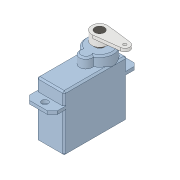
# Autodesk Inventor part: CW
Saved by Autodesk Inventor 2019 (Build 230136000, 136)
## iProperties
Created: 2022-04-05
Part Number: CW
Material: Generic
Document SubType Name: Modeling
Designer: solyo
Density: 1 g/cm^3
Appearance: Default
Mass: 3.44386 g
Surface Area: 17.9461 cm^2
Volume: 3.44386 cm^3
Author: solyo
Autodesk Inventor part; units mm, degrees
ref_plane "YZ Plane" through (0, 0, 0) normal (1, 0, 0) x (0, 1, 0)
ref_plane "XZ Plane" through (0, 0, 0) normal (0, 1, 0) x (-1, 0, 0)
ref_plane "XY Plane" through (0, 0, 0) normal (0, 0, 1) x (1, 0, 0)
sketch "Sketch1" plane through (0, 0, 0) normal (0, 1, 0) x (-1, 0, 0)
  line L0 (-4.375, -10) -> (4.375, -10)
  line L1 (4.375, -10) -> (4.375, 10)
  line L2 (4.375, 10) -> (-4.375, 10)
  line L3 (-4.375, 10) -> (-4.375, -10)
  line L4 (-4.375, -10) -> (4.375, 10) construction
  line L5 (4.375, -10) -> (-4.375, 10) construction
  point P0 (0, 0)
  dimension "d0" = 8.75
  dimension "d1" = 20
  constraints: 12 end point, 2 midpoint, 2 parallel, 1 horizontal, 1 perpendicular
  measures "d0" distance of L2.end L1.end
  measures "d1" distance of L1.end L0.end
extrude "Extrusion1" add sketch "Sketch1" along normal blind 17.7
ref_plane "Work Plane1" through (0, 12.7, 0) normal (0, -1, 0) x (1, 0, 0)
sketch "Sketch2" plane through (0, 12.7, 0) normal (0, -1, 0) x (1, 0, 0)
  line L0 (4.375, -10) -> (-4.375, -10) projected
  line L1 (4.375, -10) -> (-4.375, -10) projected
  line L2 (-4.375, -10) -> (-4.375, 10) projected
  line L3 (-4.375, 10) -> (4.375, 10) projected
  line L4 (4.375, 10) -> (4.375, -10) projected
  line L5 (-4.375, 13.75) -> (4.375, 13.75)
  line L6 (4.375, 13.75) -> (4.375, -13.75)
  line L7 (4.375, -13.75) -> (-4.375, -13.75)
  line L8 (-4.375, -13.75) -> (-4.375, 13.75)
  point P0 (0, 0)
  point P1 (0, 11.75)
  point P2 (0, -11.75)
  point P3 (0, -10)
  dimension "d5" = 23.5
  dimension "d6" = 2
  dimension "d7" = 2
  dimension "d8" = 11.75
  dimension "d9" = 11.75
  constraints: 8 end point, 4 vertical alignment, 2 parallel, 1 horizontal, 1 midpoint, 1 perpendicular
  measures "d5" distance of point (0, -11.75) point (0, 11.75)
  measures "d6" distance from line of point (0, -11.75) L7
  measures "d7" distance from line of L5 point (0, 11.75)
  measures "d8" distance of point (0, 0) point (0, -11.75)
  measures "d9" distance of point (0, 0) point (0, 11.75)
extrude "Extrusion2" add sketch "Sketch2" against normal blind 1 contours L6 L7 L8 L0 | L3 L8 L5 L6
chamfer "Chamfer1" distance 1.5 angle 45 4 edges at (4.375, 13.2, 13.75) (-4.375, 13.2, 13.75) (4.375, 13.2, -13.75) (-4.375, 13.2, -13.75)
hole "Hole1" at (0, 12.7, 11.75) at (0, 12.7, -11.75) direction (0, 1, 0) diameter 2 end through all
sketch "Sketch3" plane through (0, 17.7, 0) normal (0, 1, 0) x (1, 0, 0)
  circle A0 centre (0, 5.625) radius 4.375
  circle A1 centre (0, 1.25) radius 2
  line L0 (4.375, 10) -> (-4.375, 10) projected
  line L1 (-4.375, 10) -> (-4.375, -10) projected
  line L2 (-4.375, -10) -> (4.375, -10) projected
  line L3 (4.375, -10) -> (4.375, 10) projected
  circle A2 centre (0, 11.75) radius 1 projected
  point P0 (0, 0)
  dimension "d23" = 4
  constraints: 3 vertical alignment, 1 centre point, 1 horizontal, 1 vertical, 2 other
  measures "d23" diameter of A1
extrude "Extrusion3" add sketch "Sketch3" along normal blind 3.15 contours A0 A1 | A1 A0 | A0 A1
chamfer "Chamfer2" distance 0.5 angle 45 22 edges at (4.375, 15.7, 10) (-4.375, 15.7, 10) (-4.375, 6.35, 10) (4.375, 6.35, 10) (4.375, 6.35, -10) (4.375, 15.7, -10) (-4.375, 15.7, -10) (-4.375, 6.35, -10) (4.375, 17.7, 2.1875) (4.375, 17.7, -7.8125) (0, 13.7, -13.75) (-4.375, 17.7, 2.1875) (0, 17.7, 10) (4.375, 0, 0) (0, 0, 10) (-4.375, 0, 0) (0, 0, -10) (0, 20.85, 0.75) (0, 20.85, -10) (-4.375, 17.7, -7.8125) (-2.1875, 17.7, -10) (2.1875, 17.7, -10)
sketch "Sketch4" plane through (0, 20.85, 0) normal (0, 1, 0) x (1, 0, 0)
  arc A0 (1.3112, 1.9786) -> (-1.3112, 1.9786) centre (0, 5.625) ccw projected
  arc A1 (-1.3112, 1.9786) -> (1.3112, 1.9786) centre (0, 1.25) ccw projected
  circle A2 centre (0, 5.625) radius 1.5
  point P0 (0, 0)
  dimension "d31" = 3
  constraints: 1 centre point, 1 coincident
  measures "d31" diameter of A2
extrude "Extrusion4" add sketch "Sketch4" along normal blind 4 separate body contours A2
sketch "Sketch5" plane through (0, 24.85, -5.625) normal (0, 1, 0) x (1, 0, 0)
  circle A0 centre (0, 0) radius 1.5 projected
  arc A1 (2.4804, -0.3125) -> (-2.4804, -0.3125) centre (0, 0) ccw
  arc A2 (-1.4882, -8.1875) -> (1.4882, -8.1875) centre (0, -8) ccw
  line L0 (0, 0) -> (0, -23.0881) construction
  line L1 (0, -8) -> (0, 0) construction
  line L2 (1.4882, -8.1875) -> (2.4804, -0.3125)
  line L3 (-1.4882, -8.1875) -> (-2.4804, -0.3125)
  circle A3 centre (0, -8) radius 0.5
  point P0 (0, -5.625)
  dimension "d34" = 5
  dimension "d35" = 3
  dimension "d36" = 8
  dimension "d38" = 1
  constraints: 8 end point, 4 point on circle, 4 tangent, 3 centre point, 2 coincident, 2 vertical
  measures "d34" diameter of A1
  measures "d35" diameter of A2
  measures "d36" distance of A0.centre L1.start
  measures "d38" diameter of A3
extrude "Extrusion5" add sketch "Sketch5" against normal blind 1 separate body
sketch "Sketch6" plane through (0, 23.85, -5.625) normal (0, -1, 0) x (1, 0, 0)
  circle A0 centre (0, 0) radius 1.5 projected
  circle A1 centre (0, 0) radius 1.5 projected
  circle A2 centre (0, 8) radius 0.5 projected
  line L0 (1.4882, 8.1875) -> (2.4804, 0.3125) projected
  arc A3 (-2.4804, 0.3125) -> (2.4804, 0.3125) centre (0, 0) ccw projected
  line L1 (-2.4804, 0.3125) -> (-1.4882, 8.1875) projected
  arc A4 (1.4882, 8.1875) -> (-1.4882, 8.1875) centre (0, 8) ccw projected
  circle A5 centre (0, 0) radius 2.5
  point P0 (0, 5.625)
  constraints: 1 centre point, 1 coincident, 1 concentric
extrude "Extrusion6" add sketch "Sketch6" along normal blind 2 contours A3 A5 bodies 3
move or copy body "Rotate1" bodies to move or copy 3 copy no rotation origin (0, 0, 0) rotation axis (0, 1, 0) rotation angle 90 translate (5.625, 0, -5.625)
ref_plane "center plane" through (0, 8.85, 0) normal (0, 1, 0) x (1, 0, 0)
equation "\"d8\" = d9"
equation "\"d43\" = Angle"
equation "\"Angle\" = 90deg"
